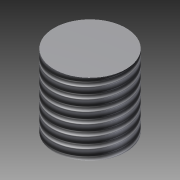
# Autodesk Inventor part: Pusher.Socketscrew
Saved by Autodesk Inventor 2011 (Build 150239000, 239)
## iProperties
Created: 2011-04-01
Part Number: Pusher.Socketscrew
Document SubType Name: Modeling
Designer: Rob
Density: 1 g/cm^3
Author: Rob
Autodesk Inventor part; units mm, degrees
ref_plane "YZ Plane" through (0, 0, 0) normal (1, 0, 0) x (0, 1, 0)
ref_plane "XZ Plane" through (0, 0, 0) normal (0, 1, 0) x (-1, 0, 0)
ref_plane "XY Plane" through (0, 0, 0) normal (0, 0, 1) x (1, 0, 0)
sketch "Sketch1" plane through (0, 0, 0) normal (0, 0, 1) x (1, 0, 0)
  circle A0 centre (0, 0) radius 5
  dimension "d0" = 10
  constraints: 1 centre point, 1 coincident
  measures "d0" diameter of A0
extrude "Extrusion1" add sketch "Sketch1" along normal blind 10
thread "Thread1" size "M10x1.5" class "6g" standard "ANSI Metric M Profile" full length
sketch "Sketch2" plane through (0, 0, 0) normal (0, 0, -1) x (-1, 0, 0)
  circle A0 centre (0, 0) radius 5 projected
  circle A1 centre (0, 0) radius 2.5
  line L0 (-1.8795, -2.5) -> (1.9053, -2.5)
  line L1 (1.2253, -2.8777) -> (3.1177, 0.4)
  line L2 (3.1048, -0.3777) -> (1.2124, 2.9)
  line L3 (1.8795, 2.5) -> (-1.9053, 2.5)
  line L4 (-1.2253, 2.8777) -> (-3.1177, -0.4)
  line L5 (-3.1048, 0.3777) -> (-1.2124, -2.9)
  line L6 (-1.4434, 2.5) -> (1.4434, 2.5)
  line L7 (1.4434, 2.5) -> (2.8868, 0)
  line L8 (2.8868, 0) -> (1.4434, -2.5)
  line L9 (1.4434, -2.5) -> (-1.4434, -2.5)
  line L10 (-1.4434, -2.5) -> (-2.8868, 0)
  line L11 (-2.8868, 0) -> (-1.4434, 2.5)
  dimension "d5" = 5
  dimension "d8" = 360
  constraints: 24 end point, 12 point on line, 1 centre point, 1 coincident, 1 collinear, 1 horizontal, 19 other
  measures "d5" diameter of A1
extrude "Extrusion2" cut sketch "Sketch2" against normal blind 5 contours A1 | A1 L2 L1 | A1 L3 L2 | L1 L0 A1 | A1 L4 L3 | L0 L5 A1 | A1 L5 L4
body "Solid1"
